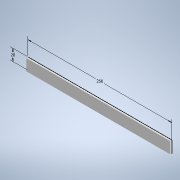
# Autodesk Inventor part: Lateral_Carril
Saved by Autodesk Inventor 2022 (Build 260153000, 153)
## iProperties
Created: 2022-01-30
Part Number: Lateral_Carril
Material: Generic
Document SubType Name: Modeling
Designer: katha
Density: 1 g/cm^3
Appearance: Default
Author: katha
Autodesk Inventor part; units mm, degrees
ref_plane "YZ Plane" through (0, 0, 0) normal (1, 0, 0) x (0, 1, 0)
ref_plane "XZ Plane" through (0, 0, 0) normal (0, 1, 0) x (-1, 0, 0)
ref_plane "XY Plane" through (0, 0, 0) normal (0, 0, 1) x (1, 0, 0)
sketch "Sketch1" plane through (0, 0, 0) normal (0, 0, 1) x (1, 0, 0)
  line L0 (125, -10) -> (-125, -10)
  line L1 (-125, -10) -> (-125, 10)
  line L2 (-125, 10) -> (125, 10)
  line L3 (125, 10) -> (125, -10)
  line L4 (125, -10) -> (-125, 10) construction
  line L5 (-125, -10) -> (125, 10) construction
  point P0 (0, 0)
  dimension "d0" = 250
  dimension "d1" = 20
  constraints: 12 end point, 2 midpoint, 2 parallel, 1 horizontal, 1 perpendicular
  measures "d0" distance of L1.end L2.end
  measures "d1" distance of L0.end L1.end
extrude "Extrusion1" add sketch "Sketch1" along normal blind 3
sketch "Sketch3" plane through (0, 0, 3) normal (0, 0, 1) x (1, 0, 0)
  line L0 (125, 10) -> (-125, 10) projected
  point P0 (0, 0)
  point P1 (0, 1.25)
  dimension "d12" = 8.75
  constraints: 1 vertical alignment
  measures "d12" distance from line of L0 point (0, 1.25)
hole "Hole2" at (0, 1.25, 3) direction (0, 0, -1) diameter 5 end through all
body "Solid1"
